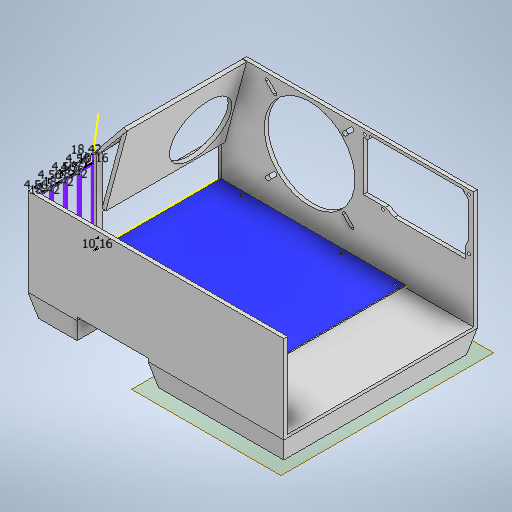
# Autodesk Inventor part: matx-arc-case-r2
Saved by Autodesk Inventor 2025 (Build 290162000, 162)
## iProperties
Created: 2024-07-20
Part Number: matx-arc-case-r2
Material: Generic
Document SubType Name: Modeling
Designer: admin
Density: 1 g/cm^3
Appearance: Default
Author: admin
Autodesk Inventor part; units mm, degrees
ref_plane "YZ Plane" through (0, 0, 0) normal (1, 0, 0) x (0, 1, 0)
ref_plane "XZ Plane" through (0, 0, 0) normal (0, 1, 0) x (-1, 0, 0)
ref_plane "XY Plane" through (0, 0, 0) normal (0, 0, 1) x (1, 0, 0)
sketch "Sketch2" plane through (0, 0, 0) normal (0, 1, 0) x (-1, 0, 0)
  line L0 (0, 0) -> (0, -243.84)
  line L1 (0, -243.84) -> (243.84, -243.84)
  line L2 (243.84, -243.84) -> (243.84, 0)
  line L3 (243.84, 0) -> (0, 0)
  line L4 (243.84, 0) -> (233.68, 0)
  line L5 (233.68, 0) -> (6.35, 0)
  line L6 (233.68, 0) -> (78.74, 0)
  line L7 (233.68, -243.84) -> (210.82, -243.84)
  line L8 (233.68, 0) -> (233.68, -243.84)
  line L9 (243.84, -243.84) -> (243.84, -85.09)
  line L10 (6.35, 0) -> (6.35, -243.84)
  line L11 (78.74, 0) -> (78.74, -243.84)
  line L12 (243.84, -85.09) -> (243.84, -31.85)
  line L13 (78.74, -31.85) -> (78.74, -77.57)
  line L14 (78.74, 0) -> (78.74, -34.29)
  line L15 (78.74, -34.29) -> (78.74, -13.97)
  line L16 (78.74, -34.29) -> (78.74, -80.01)
  circle A0 centre (78.74, -80.01) radius 2
  circle A1 centre (78.74, -34.29) radius 2
  circle A2 centre (78.74, -13.97) radius 2
  circle A3 centre (6.35, -80.01) radius 2
  line L17 (78.74, -34.29) -> (78.74, -237.49)
  circle A4 centre (78.74, -237.49) radius 2
  circle A5 centre (6.35, -237.49) radius 2
  circle A6 centre (210.82, -237.49) radius 2
  circle A7 centre (233.68, -34.29) radius 2
  circle A8 centre (233.68, -80.01) radius 2
  dimension "d79" = 243.84
  dimension "d80" = 243.84
  dimension "d81" = 10.16
  dimension "d82" = 227.33
  dimension "d83" = 154.94
  dimension "d84" = 22.86
  dimension "d85" = 158.75
  dimension "d92" = 34.29
  dimension "d93" = 20.32
  dimension "d94" = 45.72
  dimension "d95" = 203.2
  constraints: 36 end point, 17 point on line, 9 centre point, 4 coincident, 4 perpendicular, 2 vertical, 1 parallel
  measures "d79" distance of L0.start L0.end
  measures "d80" distance of L0.end L1.end
  measures "d81" distance of L2.end L4.end
  measures "d82" distance of L4.end L5.end
  measures "d83" distance of L4.end L6.end
  measures "d84" distance of L7.start L7.end
  measures "d85" distance of L1.end L9.end
  measures "d92" distance of L6.end L14.end
  measures "d93" distance of L14.end L15.end
  measures "d94" distance of L14.end L16.end
  measures "d95" distance of L17.start L17.end
extrude "Extrusion1" add sketch "Sketch2" along normal blind 1.5 contours L3 L10 A3 A5 L1 L0 | L3 L11 A2 A1 A0 A4 L1 L10 A5 A3 | L3 L8 A7 A8 L1 L11 A4 A0 A1 A2 | L3 L2 L1 L8 A8 A7
sketch "Sketch4" plane through (-243.84, 0, -243.84) normal (-1, 0, 0) x (0, 0, 1)
  line L0 (0.0105, -0.4083) -> (0.0105, -1.9083)
  line L1 (243.84, 0) -> (0, 0) projected
  line L2 (0.0105, -1.9083) -> (-1.25, -1.9083)
  line L3 (-1.25, -1.9083) -> (-1.25, 42.5417)
  line L4 (-1.25, -1.9083) -> (43.2, -1.9083) construction
  line L5 (-1.25, 42.5417) -> (157.5, 42.5417)
  line L6 (157.5, 42.5417) -> (157.5, -1.9083)
  line L7 (-1.25, -1.9083) -> (-1.25, -6.0083)
  line L8 (-1.25, -6.0083) -> (157.5, -6.0083)
  line L9 (-1.25, -6.0083) -> (-5.35, -6.0083)
  line L10 (-5.35, -6.0083) -> (-5.35, 42.5417)
  line L11 (-5.35, 42.5417) -> (-5.35, 46.6417)
  line L12 (-5.35, 46.6417) -> (157.5, 46.6417)
  line L13 (157.5, 46.6417) -> (161.6, 46.6417)
  line L14 (161.6, 46.6417) -> (161.6, -1.9083)
  line L15 (161.6, -6.0083) -> (157.5, -6.0083)
  line L16 (161.6, -6.0083) -> (161.6, -1.9083)
  line L17 (0.0105, -1.9083) -> (157.5, -1.9083)
  line L18 (161.6, -6.0083) -> (243.84, -6.0083)
  line L19 (161.6, -6.0083) -> (161.6, 9.1917)
  line L20 (161.6, 9.1917) -> (243.84, 9.1917)
  line L21 (243.84, 9.1917) -> (243.84, -6.0083)
  line L22 (157.5, 42.5417) -> (164.5, 42.5417)
  line L23 (164.5, 42.5417) -> (164.5, 9.1917)
  line L24 (164.5, 42.5417) -> (164.5, 46.6417)
  line L25 (164.5, 46.6417) -> (161.6, 46.6417)
  line L26 (164.5, 9.1917) -> (164.5, 110.1917)
  line L27 (164.5, 110.1917) -> (243.84, 110.1917)
  line L28 (243.84, 110.1917) -> (243.84, 9.1917)
  line L29 (157.5, 46.6417) -> (157.5, 110.1917)
  line L30 (250.84, 110.1917) -> (250.84, -6.0083)
  line L31 (250.84, -6.0083) -> (243.84, -6.0083)
  line L32 (243.84, 110.1917) -> (250.84, 110.1917)
  line L33 (157.5, 110.1917) -> (164.5, 110.1917)
  line L34 (157.5, 46.6417) -> (157.5, 132.6417)
  line L35 (157.5, 132.6417) -> (7.5, 132.6417)
  line L36 (7.5, 132.6417) -> (7.5, 46.6417)
  dimension "d98" = 1.5
  dimension "d103" = 44.45
  dimension "d104" = 90
  dimension "d105" = 158.75
  dimension "d106" = 4.1
  dimension "d107" = 4.1
  dimension "d108" = 4.1
  dimension "d109" = 4.1
  dimension "d110" = 15.2
  dimension "d111" = 7
  dimension "d112" = 101
  dimension "d165" = 86
  dimension "d166" = 150
  constraints: 72 end point, 16 perpendicular, 14 point on line, 4 vertical, 3 horizontal, 2 collinear, 2 parallel
  measures "d98" distance of L0.start L0.end
  measures "d103" distance of L2.end L3.end
  measures "d104" angle of L4 L3
  measures "d105" distance of L3.end L5.end
  measures "d106" distance of L2.end L7.end
  measures "d107" distance of L7.end L9.end
  measures "d108" distance of L10.end L11.end
  measures "d109" distance of L12.end L13.end
  measures "d110" distance of L15.start L19.end
  measures "d111" distance of L5.end L22.end
  measures "d112" distance of L23.end L26.end
  measures "d165" distance of L12.end L34.end
  measures "d166" distance of L34.end L35.end
extrude "Extrusion2" add sketch "Sketch4" along normal blind 5 contours L21 L18 L16 L14 L1 | L1 L14 L20 L21 | L21 L28 L32 L30 L31 | L14 L16 L15 L8 L7 L2 L17 L6 L1 | L1 L6 L22 L14 | L14 L22 L23 L20 | L5 L3 L7 L9 L10 L11 L12 L13 L14 L22 | L14 L25 L24 L22 | L26 L25 L13 L29 L33
sketch "Sketch5" plane through (-243.84, 0, -243.84) normal (1, 0, 0) x (0, 0, -1)
  line L0 (5.35, -6.0083) -> (-250.84, -6.0083) projected
  line L1 (-250.84, -6.0083) -> (5.35, -6.0083)
  line L2 (5.35, -6.0083) -> (5.35, -1.9083)
  line L3 (5.35, -1.9083) -> (-250.84, -1.9083)
  line L4 (-157.5, -1.9083) -> (1.25, -1.9083) projected
  line L5 (-250.84, -1.9083) -> (-250.84, -6.0083)
  point P0 (-243.84, 0)
  constraints: 8 end point, 2 collinear, 2 perpendicular
extrude "Extrusion3" add sketch "Sketch5" along normal blind 60
sketch "Sketch6" plane through (-248.84, -1.9083, -86.34) normal (0, 1, 0) x (1, 0, 0)
  circle A0 centre (15.16, -52.05) radius 2 projected
  circle A1 centre (15.16, -52.05) radius 2
  circle A2 centre (15.16, -6.33) radius 2 projected
  circle A3 centre (15.16, -6.33) radius 2
  circle A4 centre (37.9882, 151.128) radius 2.0223
  point P0 (248.84, -86.34)
  constraints: 3 centre point, 2 coincident
extrude "Extrusion4" cut sketch "Sketch6" against normal blind 28.25
ref_plane "Work Plane1" through (-248.84, -36.0083, -249.19) normal (0, -1, 0) x (1, 0, 0)
sketch "Sketch7" plane through (-248.84, -36.0083, -249.19) normal (0, -1, 0) x (1, 0, 0)
  line L0 (65, 256.19) -> (65, 0) projected
  line L1 (65, 256.19) -> (65, 249.19)
  line L2 (7, 249.19) -> (7, 7)
  line L3 (7, 7) -> (58, 7)
  line L4 (58, 7) -> (58, 249.19)
  line L5 (58, 249.19) -> (7, 249.19)
  line L6 (5, 249.19) -> (248.84, 249.19) projected
  dimension "d122" = 7
  constraints: 10 end point, 2 perpendicular, 1 collinear, 1 point on line
  measures "d122" distance of L1.end L4.end
loft "Loft1" add profiles "Sketch7" section 2 edges at (-216.34, -6.0083, 7) (-248.84, -6.0083, -121.095) (-216.34, -6.0083, -249.19) (-183.84, -6.0083, -121.095)
ref_plane "Work Plane2" through (0.16, 0, -243.84) normal (1, 0, 0) x (0, 0, -1)
sketch "Sketch8" plane through (0.16, 0, -243.84) normal (1, 0, 0) x (0, 0, -1)
  line L0 (5.35, -1.9083) -> (-250.84, -1.9083) projected
  line L1 (-250.84, -1.9083) -> (5.35, -1.9083)
  line L2 (5.35, -6.0083) -> (-250.84, -6.0083) projected
  line L3 (5.35, -1.9083) -> (5.35, -6.0083)
  line L4 (5.35, -6.0083) -> (-250.84, -6.0083)
  line L5 (-250.84, -6.0083) -> (-250.84, -1.9083)
  point P0 (-243.84, 0)
  constraints: 8 end point, 3 perpendicular, 1 horizontal
extrude "Extrusion5" add sketch "Sketch8" along normal blind 90 and the other way blind 90
sketch "Sketch10" plane through (-248.84, -1.9083, -86.34) normal (0, 1, 0) x (1, 0, 0)
  line L0 (5, 158.75) -> (5, 162.85) projected
  line L1 (166, 169.85) -> (165.809, 162.6689) projected
  line L2 (5, 162.85) -> (159, 162.85)
  line L3 (159, 162.85) -> (159, 158.35)
  line L4 (159, 158.35) -> (5, 158.35)
  line L5 (5, 158.35) -> (5, 162.85)
  point P0 (248.84, -86.34)
  point P1 (244.5, 158.35)
  dimension "d142" = 4.5
  constraints: 8 end point, 3 perpendicular, 1 horizontal, 1 other
  measures "d142" distance of L2.end L3.end
extrude "Extrusion6" [suppressed]
sketch "Sketch11" plane through (-183.84, -1.9083, -244.69) normal (0, 0, 1) x (1, 0, 0)
  point P0 (183.84, 1.9083)
sketch "Sketch13" plane through (-183.84, -6.0083, -249.19) normal (0, 0, -1) x (-1, 0, 0)
  line L0 (-74.6961, 108.9977) -> (-74.6961, 18.9977)
  line L1 (-74.6961, 18.9977) -> (15.3039, 18.9977)
  line L2 (15.3039, 18.9977) -> (15.3039, 108.9977)
  line L3 (58.6377, 116.2) -> (-81.3623, 116.2) projected
  line L4 (15.3039, 108.9977) -> (-74.6961, 108.9977)
  point P0 (-183.84, 6.0083)
  dimension "d149" = 90
  dimension "d150" = 90
  constraints: 8 end point, 3 perpendicular, 1 vertical
  measures "d149" distance of L0.start L0.end
  measures "d150" distance of L0.end L1.end
extrude "Extrusion8" cut sketch "Sketch13" against normal blind 24.5
sketch "Sketch14" plane through (90.16, -1.9083, 7) normal (0, 1, 0) x (1, 0, 0)
  line L0 (-334, 0) -> (-334, 93.34) projected
  line L1 (-180, 0) -> (0, 0) projected
  line L2 (-334, 0) -> (-180, 0)
  line L3 (-180, 0) -> (-180, 5)
  line L4 (-180, 5) -> (-334, 5)
  line L5 (-334, 5) -> (-334, 0)
  line L6 (-180, 5) -> (0, 5)
  line L7 (0, 256.19) -> (0, 0) projected
  point P0 (-90.16, 7)
  dimension "d154" = 5
  constraints: 10 end point, 3 perpendicular, 2 horizontal, 1 point on line
  measures "d154" distance of L1.start L3.end
extrude "Extrusion9" add sketch "Sketch14" along normal blind 112.1
sketch "Sketch15" plane through (-89.84, -1.9083, 2) normal (0, 0, -1) x (-1, 0, 0)
  line L0 (152.6377, 112.1) -> (12.6377, 112.1) projected
  arc A0 (12.6377, 112.1) -> (-90, 48.54) centre (12.6377, -2.5505) ccw projected
  arc A1 (12.6377, 112.1) -> (-85.9195, 56.0261) centre (12.6377, -2.5505) ccw
  arc A2 (-90, 48.54) -> (-91.2698, 0) centre (-5.2421, 22.0361) ccw projected
  arc A3 (-85.9195, 56.0261) -> (-90, -4.4678) centre (-13.3257, 20.7448) ccw
  line L1 (0, 112.1) -> (159, 112.1) projected
  line L2 (-90, -4.4678) -> (-90, 112.1)
  line L3 (0, 112.1) -> (12.6377, 112.1)
  point P0 (-89.84, 1.9083)
  point P1 (-92.4159, 38.9798)
  point P2 (-90, 45.9575)
  point P3 (-0.5912, 111.3342)
  point P4 (-85.9195, 56.0261)
  point P5 (-94.0389, 20.8167)
  constraints: 4 point on circle, 2 centre point, 2 end point, 1 collinear, 3 other
extrude "Extrusion10" [suppressed]
sketch "Sketch16" plane through (-89.84, -1.9083, 2) normal (0, 0, -1) x (-1, 0, 0)
  line L0 (12.6377, 112.1) -> (159, 112.1) projected
  line L1 (159, 112.1) -> (159, 102.1)
  line L2 (159, -4.1) -> (159, 112.1) projected
  line L3 (12.6377, 102.1) -> (12.6377, -0.0079)
  line L4 (12.6377, -0.0079) -> (12.6377, 9.9921)
  line L5 (12.6377, 9.9921) -> (149, 9.9921)
  line L6 (149, 9.9921) -> (149, 102.1)
  line L7 (149, 102.1) -> (12.6377, 102.1)
  arc A0 (-85.9195, 56.0261) -> (-90, 45.9575) centre (-13.3257, 20.7448) ccw projected
  point P0 (-89.84, 1.9083)
  dimension "d160" = 10
  constraints: 12 end point, 2 point on line, 1 horizontal, 1 perpendicular
  measures "d160" distance of L3.end L4.end
extrude "Extrusion11" [suppressed]
sketch "Sketch18" plane through (-89.84, -1.9083, -249.19) normal (0, 1, 0) x (1, 0, 0)
  line L0 (-154, 0) -> (-94, 0) projected
  line L1 (-154, 0) -> (-154, -5)
  line L2 (-154, -4.1) -> (-154, 0) projected
  line L3 (-154, -5) -> (180, -5)
  line L4 (180, 0) -> (180, -256.19) projected
  line L5 (180, -5) -> (180, 0)
  line L6 (180, 0) -> (-154, 0)
  line L7 (-154, -5) -> (-154, 0)
  point P0 (89.84, -249.19)
  dimension "d173" = 5
  constraints: 10 end point, 2 collinear, 1 parallel, 1 perpendicular, 1 point on line, 1 vertical
  measures "d173" distance of L0.start L1.end
extrude "Extrusion13" add sketch "Sketch18" along normal blind 155
sketch "Sketch19" plane through (-183.84, -6.0083, -249.19) normal (0, 0, -1) x (-1, 0, 0)
  line L0 (-274, 159.1) -> (-124, 159.1)
  line L1 (-124, 159.1) -> (-124, 73.1)
  line L2 (-124, 73.1) -> (-274, 73.1)
  line L3 (-124, 73.1) -> (-124, 79.1)
  line L4 (-124, 79.1) -> (-124, 153.1)
  circle A0 centre (-268, 85.1) radius 2
  line L5 (-268, 159.1) -> (-268, 153.1)
  circle A1 centre (-268, 153.1) radius 2
  line L6 (-274, 0) -> (-274, 159.1) projected
  line L7 (-274, 159.1) -> (-274, 73.1)
  circle A2 centre (-154, 79.1) radius 2
  circle A3 centre (-130, 153.1) radius 2
  line L8 (-274, 159.1) -> (-274, 73.1)
  line L9 (-136.2898, 155.1) -> (-136.2898, 151.1)
  line L10 (-136.2898, 151.1) -> (-132.8214, 148.8373)
  line L11 (-132.8214, 148.8373) -> (-128, 148.8373)
  line L12 (-128, 148.8373) -> (-128, 83.1)
  line L13 (-128, 83.1) -> (-157.5962, 83.1)
  line L14 (-157.5962, 83.1) -> (-162.4696, 80.5434)
  line L15 (-162.4696, 80.5434) -> (-169.0334, 77.1)
  line L16 (-169.0334, 77.1) -> (-263.6103, 77.1)
  line L17 (-263.6103, 77.1) -> (-263.6103, 92.4697)
  line L18 (-263.6103, 92.4697) -> (-268, 100.8374)
  line L19 (-268, 100.8374) -> (-268, 145.9566)
  line L20 (-268, 145.9566) -> (-261.4865, 153.1)
  line L21 (-261.4865, 153.1) -> (-261.4865, 155.1)
  line L22 (-261.4865, 155.1) -> (-136.2898, 155.1)
  point P0 (-183.84, 6.0083)
  dimension "d176" = 150
  dimension "d177" = 86
  dimension "d187" = 6
  dimension "d188" = 74
  dimension "d190" = 4
  dimension "d191" = 4
  dimension "d194" = 4
  dimension "d196" = 4
  constraints: 44 end point, 7 perpendicular, 4 centre point, 4 parallel, 3 point on line, 2 collinear, 1 coincident, 1 vertical
  measures "d176" distance of L0.start L0.end
  measures "d177" distance of L0.end L1.end
  measures "d187" distance of L1.end L3.end
  measures "d188" distance of L3.end L4.end
  measures "d190" diameter of A0
  measures "d191" diameter of A1
  measures "d194" diameter of A2
  measures "d196" diameter of A3
ref_plane "Work Plane5" through (-89.84, -36.0083, -249.19) normal (0, -1, 0) x (1, 0, 0)
sketch "Sketch21" plane through (-89.84, -36.0083, -249.19) normal (0, -1, 0) x (1, 0, 0)
  line L0 (6.9942, 7.0266) -> (172.9817, 7.0266)
  line L1 (172.9817, 7.0266) -> (172.9817, 249.19)
  line L2 (172.9817, 249.19) -> (6.9942, 249.19)
  line L3 (6.9942, 249.19) -> (6.9942, 7.0266)
  constraints: 8 end point, 1 horizontal, 1 perpendicular, 1 vertical
loft "Loft3" add profiles "Sketch21" section 2 edges at (0.16, -6.0083, -249.19) (90.16, -6.0083, -121.095) (0.16, -6.0083, 7) (-89.84, -6.0083, -121.095)
extrude "Extrusion14" cut sketch "Sketch19" against normal blind 112.1 contours A0 | A1 | A2 | A3 | L9 L10 L11 L12 L13 L14 L15 L16 L17 L18 L19 L20 L21 L22
sketch "Sketch22" plane through (-183.84, -6.0083, -249.19) normal (0, 0, -1) x (-1, 0, 0)
  line L0 (-274, 116.2) -> (60, 116.2) projected
  line L1 (-117.0064, 154.3094) -> (-117.0064, 34.3094)
  line L2 (-117.0064, 34.3094) -> (2.9936, 34.3094)
  line L3 (2.9936, 34.3094) -> (2.9936, 154.3094)
  line L4 (2.9936, 154.3094) -> (-117.0064, 154.3094)
  circle A0 centre (-57.0064, 94.3094) radius 60
  arc A1 (-115.0678, 39.7836) -> (-111.5322, 36.248) centre (-113.3, 38.0158) ccw
  arc A2 (-101.2647, 46.5156) -> (-104.8003, 50.0511) centre (-103.0325, 48.2833) ccw
  line L5 (-104.8003, 50.0511) -> (-115.0678, 39.7836)
  line L6 (-111.5322, 36.248) -> (-101.2647, 46.5156)
  arc A3 (-2.4806, 36.248) -> (1.055, 39.7836) centre (-0.7128, 38.0158) ccw
  arc A4 (-9.2125, 50.0511) -> (-12.7481, 46.5156) centre (-10.9803, 48.2833) ccw
  arc A5 (-12.7481, 142.1033) -> (-9.2125, 138.5678) centre (-10.9803, 140.3355) ccw
  arc A6 (1.055, 148.8353) -> (-2.4806, 152.3708) centre (-0.7128, 150.603) ccw
  arc A7 (-111.5322, 152.3708) -> (-115.0678, 148.8353) centre (-113.3, 150.603) ccw
  arc A8 (-104.8003, 138.5678) -> (-101.2647, 142.1033) centre (-103.0325, 140.3355) ccw
  line L7 (-111.5322, 152.3708) -> (-101.2647, 142.1033)
  line L8 (-115.0678, 148.8353) -> (-104.8003, 138.5678)
  line L9 (1.055, 148.8353) -> (-9.2125, 138.5678)
  line L10 (-2.4806, 152.3708) -> (-12.7481, 142.1033)
  line L11 (-9.2125, 50.0511) -> (1.055, 39.7836)
  line L12 (-12.7481, 46.5156) -> (-2.4806, 36.248)
  line L13 (1.055, 36.248) -> (2.9936, 34.3094)
  point P0 (-183.84, 6.0083)
  dimension "d200" = 120
  dimension "d201" = 120
  dimension "d202" = 5
  dimension "d203" = 5
  dimension "d204" = 5
  dimension "d205" = 5
  dimension "d206" = 5
  dimension "d207" = 5
  dimension "d208" = 5
  constraints: 26 end point, 17 point on circle, 9 centre point, 7 tangent, 5 point on line, 4 perpendicular, 2 parallel, 1 vertical
  measures "d200" distance of L1.start L1.end
  measures "d201" distance of L1.end L2.end
  measures "d202" diameter of A1
  measures "d203" diameter of A2
  measures "d204" diameter of A3
  measures "d205" diameter of A4
  measures "d206" diameter of A5
  measures "d207" diameter of A6
  measures "d208" diameter of A7
extrude "Extrusion15" cut sketch "Sketch22" against normal blind 112.1 contours A0 L0 | L0 A0 | L5 A2 L6 A1 | L12 A4 L11 A3 | L10 A6 L9 A5 | L7 A8 L8 A7
chamfer "Chamfer1" distance 28.5 angle 75 1 edges at (-243.84, 153.0917, -246.69) measured on face at (-243.34, 153.0917, -246.69)
sketch "Sketch23" plane through (-215.34, 153.0917, -249.19) normal (-0.9659258, 0.258819, 0) x (0, 0, 1)
  line L0 (162.85, -110.1991) -> (5, -110.1991) projected
  line L1 (5, -110.1991) -> (162.85, -110.1991)
  line L2 (162.85, -110.1991) -> (162.85, -0.0316)
  line L3 (162.85, -0.0316) -> (5, -0.0316)
  line L4 (5, -0.0316) -> (5, -110.1991)
  point P0 (249.19, -92.1411)
  point P1 (162.85, -110.1991)
  constraints: 8 end point, 2 horizontal, 2 perpendicular
extrude "Extrusion16" add sketch "Sketch23" against normal blind 5
sketch "Sketch24" plane through (-243.84, 0, -243.84) normal (1, 0, 0) x (0, 0, -1)
  point P0 (-243.84, 0)
loft "Loft4" add section 1 edges at (-243.84, 110.1917, -82.84) (-246.34, 110.1917, -86.34) (-248.84, 110.1917, -82.84) (-246.34, 110.1917, -79.34) section 2 edges at (-215.3482, 153.0611, -165.265) (-212.9334, 152.4141, -86.34) (-210.5186, 151.767, -165.265) (-212.9334, 152.4141, -244.19)
sketch "Sketch25" plane through (-243.8616, 46.6475, -244.19) normal (-0.9659258, 0.258819, 0) x (0, 0, 1)
  line L0 (3.3975, 2.9257) -> (3.3975, 82.9257)
  line L1 (3.3975, 82.9257) -> (83.3975, 82.9257)
  line L2 (83.3975, 82.9257) -> (83.3975, 2.9257)
  line L3 (83.3975, 2.9257) -> (3.3975, 2.9257)
  circle A0 centre (43.3975, 42.9257) radius 40
  point P0 (244.19, 18.0581)
  dimension "d220" = 80
  dimension "d221" = 80
  constraints: 8 end point, 3 perpendicular, 1 centre point, 1 vertical
  measures "d220" distance of L0.start L0.end
  measures "d221" distance of L0.end L1.end
extrude "Extrusion17" cut sketch "Sketch25" against normal blind 5 contours A0
sketch "Sketch26" plane through (-248.84, 0, -243.84) normal (-1, 0, 0) x (0, 0, 1)
  line L0 (164.5, 110.1917) -> (157.5, 151.767) projected
  line L1 (164.5, 110.1917) -> (182.92, 110.1917)
  line L2 (182.92, 110.1917) -> (201.34, 110.1917)
  line L3 (201.34, 110.1917) -> (219.76, 110.1917)
  line L4 (219.76, 110.1917) -> (238.18, 110.1917)
  line L5 (238.18, 110.1917) -> (243.84, 110.1917)
  line L6 (173.71, 110.1917) -> (173.71, 100.0317)
  line L7 (173.71, 100.0317) -> (238.18, 100.0317)
  line L8 (238.18, 100.0317) -> (238.18, 9.1917)
  line L9 (238.18, 9.1917) -> (164.5, 9.1917)
  line L10 (164.5, 9.1917) -> (164.5, 110.1917)
  line L11 (173.71, 100.0317) -> (164.5, 100.0317)
  line L12 (182.92, 105.6317) -> (182.92, 9.1917)
  line L13 (219.76, 105.6317) -> (219.76, 9.1917)
  line L14 (201.34, 105.6317) -> (201.34, 9.1917)
  line L15 (182.92, 110.1917) -> (187.48, 110.1917)
  line L16 (187.48, 110.1917) -> (187.48, 105.6317)
  line L17 (187.48, 105.6317) -> (182.92, 105.6317)
  line L18 (201.34, 110.1917) -> (205.9, 110.1917)
  line L19 (205.9, 110.1917) -> (205.9, 105.6317)
  line L20 (205.9, 105.6317) -> (201.34, 105.6317)
  line L21 (219.76, 110.1917) -> (224.32, 110.1917)
  line L22 (224.32, 110.1917) -> (224.32, 105.6317)
  line L23 (224.32, 105.6317) -> (219.76, 105.6317)
  line L24 (238.18, 100.0317) -> (238.18, 105.6317)
  line L25 (238.18, 110.1917) -> (242.74, 110.1917)
  line L26 (242.74, 110.1917) -> (242.74, 105.6317)
  line L27 (242.74, 105.6317) -> (238.18, 105.6317)
  line L28 (164.5, 9.1917) -> (164.5, -0.9683)
  line L29 (161.83, -1.9083) -> (165.83, -1.9083) projected
  line L30 (164.5, -0.9683) -> (182.92, -0.9683)
  line L31 (157.5, 1.5) -> (243.84, 1.5) projected
  line L32 (182.92, -0.9683) -> (182.92, 9.1917)
  line L33 (166.6305, 97.538) -> (180.5123, 97.538)
  line L34 (180.5123, 97.538) -> (180.5123, 15.0894)
  line L35 (180.5123, 15.0894) -> (166.6305, 15.0894)
  line L36 (166.6305, 15.0894) -> (166.6305, 97.538)
  line L37 (185.2, 97.538) -> (199.0283, 97.538)
  line L38 (199.0283, 97.538) -> (199.0283, 15.0894)
  line L39 (199.0283, 15.0894) -> (185.2, 15.0894)
  line L40 (185.2, 15.0894) -> (185.2, 97.538)
  line L41 (203.62, 97.538) -> (217.5142, 97.538)
  line L42 (217.5142, 97.538) -> (217.5142, 15.0894)
  line L43 (217.5142, 15.0894) -> (203.62, 15.0894)
  line L44 (203.62, 15.0894) -> (203.62, 97.538)
  line L45 (222.04, 97.538) -> (235.6375, 97.538)
  line L46 (235.6375, 97.538) -> (235.6375, 15.0894)
  line L47 (235.6375, 15.0894) -> (222.04, 15.0894)
  line L48 (222.04, 15.0894) -> (222.04, 97.538)
  circle A0 centre (173.5714, 9.1917) radius 9.1324
  circle A1 centre (192.1142, 9.1917) radius 9.1324
  circle A2 centre (210.5671, 9.1917) radius 9.1324
  circle A3 centre (228.8388, 9.1917) radius 9.1324
  line L49 (182.92, -0.9683) -> (238.18, -0.9683)
  line L50 (-0.35, -1.9083) -> (245.84, -1.9083) projected
  line L51 (238.18, -0.9683) -> (238.18, 9.1917)
  line L52 (201.34, 9.1917) -> (201.34, -0.9683)
  line L53 (219.76, 9.1917) -> (219.76, -0.9683)
  dimension "d224" = 18.42
  dimension "d225" = 18.42
  dimension "d226" = 18.42
  dimension "d227" = 18.42
  dimension "d228" = 10.16
  dimension "d229" = 4.56
  dimension "d230" = 4.56
  dimension "d231" = 4.56
  dimension "d232" = 4.56
  dimension "d233" = 4.56
  dimension "d235" = 10.16
  constraints: 98 end point, 20 point on line, 16 perpendicular, 10 parallel, 6 vertical, 5 horizontal, 4 centre point, 1 midpoint, 10 other
  measures "d224" distance of L0.start L1.end
  measures "d225" distance of L1.end L2.end
  measures "d226" distance of L2.end L3.end
  measures "d227" distance of L3.end L4.end
  measures "d228" distance of L6.start L6.end
  measures "d229" distance of L1.end L15.end
  measures "d230" distance of L15.end L16.end
  measures "d231" distance of L2.end L18.end
  measures "d232" distance of L3.end L21.end
  measures "d233" distance of L4.end L25.end
  measures "d235" distance of L10.start L28.end
body "Solid1"
